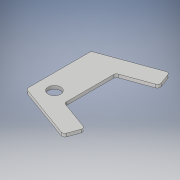
# Autodesk Inventor part: controller
Saved by Autodesk Inventor 2019 (Build 230136000, 136)
## iProperties
Created: 2019-06-18
Part Number: controller
Material: Generic
Document SubType Name: Modeling
Designer: abdel
Density: 1 g/cm^3
Appearance: Default
Author: abdel
Autodesk Inventor part; units mm, degrees
ref_plane "YZ Plane" through (0, 0, 0) normal (1, 0, 0) x (0, 1, 0)
ref_plane "XZ Plane" through (0, 0, 0) normal (0, 1, 0) x (-1, 0, 0)
ref_plane "XY Plane" through (0, 0, 0) normal (0, 0, 1) x (1, 0, 0)
sketch "Sketch1" plane through (0, 0, 0) normal (0, 1, 0) x (-1, 0, 0)
  circle A0 centre (34.925, 5.5508) radius 13.97
  line L0 (69.85, 28.9263) -> (69.85, -106.7248)
  line L1 (0, -91.6029) -> (0, 13.8044)
  line L2 (-4.1782, 19.7715) -> (-65.6375, 42.1409)
  line L3 (-4.1782, -97.57) -> (-65.6375, -119.9394)
  line L4 (65.6718, 34.8933) -> (-52.6066, 77.9431)
  line L5 (65.6718, -112.6918) -> (-52.6066, -155.7416)
  line L6 (-69.4327, 50.2797) -> (-60.7454, 74.1479)
  line L7 (-69.4327, -128.0782) -> (-60.7454, -151.9464)
  arc A1 (-69.4327, 50.2797) -> (-65.6375, 42.1409) centre (-63.4657, 48.1079) ccw
  arc A2 (-52.6066, 77.9431) -> (-60.7454, 74.1479) centre (-54.7784, 71.9761) ccw
  arc A3 (-65.6375, -119.9394) -> (-69.4327, -128.0782) centre (-63.4657, -125.9064) ccw
  arc A4 (-60.7454, -151.9464) -> (-52.6066, -155.7416) centre (-54.7784, -149.7746) ccw
  arc A5 (69.85, 28.9263) -> (65.6718, 34.8933) centre (63.5, 28.9263) ccw
  arc A6 (65.6718, -112.6918) -> (69.85, -106.7248) centre (63.5, -106.7248) ccw
  arc A7 (-4.1782, -97.57) -> (0, -91.6029) centre (-6.35, -91.6029) ccw
  arc A8 (0, 13.8044) -> (-4.1782, 19.7715) centre (-6.35, 13.8044) ccw
  point P0 (0, 0)
  point P1 (0, 18.2508)
  point P2 (0, -96.0492)
  point P3 (-71.6046, 44.3127)
  point P4 (-71.6046, -122.1112)
  point P5 (69.85, 33.3726)
  point P6 (-58.5736, 80.115)
  point P7 (69.85, -111.1711)
  point P8 (-58.5736, -157.9135)
  dimension "d4" = 27.94
  dimension "d9" = 114.3
  dimension "d10" = 76.2
  dimension "d11" = 110
  dimension "d12" = 76.2
  dimension "d13" = 110
  dimension "d14" = 38.1
  dimension "d15" = 38.1
  dimension "d17" = 34.925
  dimension "d18" = 12.7
  dimension "d21" = 6.35
  dimension "d22" = 6.35
  dimension "d23" = 69.85
  constraints: 16 end point, 16 point on circle, 16 point on line, 16 tangent, 9 centre point, 6 equal radius, 3 parallel
  measures "d4" diameter of A0
  measures "d9" distance of point (0, -96.049) point (0, 18.251)
  measures "d10" distance of point (0, 18.251) point (-71.605, 44.313)
  measures "d11" angle of L2 L1
  measures "d12" distance of point (0, -96.049) point (-71.605, -122.111)
  measures "d13" angle of L3 L1
  measures "d14" distance between parallel lines of L2 L4
  measures "d15" distance between parallel lines of L3 L5
  measures "d17" distance from line of L1 A0.centre
  measures "d18" vertical distance of point (0, 18.251) A0.centre
  measures "d21" radius of A1
  measures "d22" radius of A5
  measures "d23" distance between parallel lines of L0 L1
extrude "Extrusion1" add sketch "Sketch1" along normal blind 7.112
body "Solid1"
